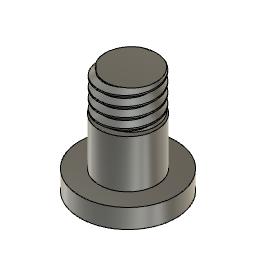
axle wheel right rear (Autodesk Fusion 360 design; units mm, degrees)
Autodesk Fusion 360 part; units mm, degrees
mesh "Mesh1" [no effect] in component "axle wheel right rear"
sketch "axle wheel right rear" plane through (0, 0, 0) normal (0, 0, 1) x (1, 0, 0) in component "axle wheel right rear"
  circle A0 centre (0, 0) radius 5
  circle A1 centre (0, 0) radius 3.0008
  constraint concentric A0 A1
extrude "Extrude1" add sketch "axle wheel right rear" along normal blind 2 contours A0 | A1 makes body 1 in component "axle wheel right rear"
extrude "Extrude2" add sketch "axle wheel right rear" along normal blind 7 contours A1 bodies 1 in component "axle wheel right rear"
extrude "Extrude3" add 1 faces at (0.1785, 0.782, 7) along direction (0, 0, 1) blind 4 separate body on bodies 1 makes body 2 in component "axle wheel right rear"
thread "Thread1" "ISO Metric profile 6.0 M6x1 6g" major diameter 5.884 minor diameter 4.7435 pitch 1 angle 60 modelled right hand crest width 0.1444 on face at (2.997, -0.1496, 9.6667) crest through (2.942, 0, 6.75) on bodies 2 in component "axle wheel right rear"
combine "Combine1" operation add target body 1 tool bodies 2 in component "axle wheel right rear"
component "axle wheel right rear" placed x (1, 0, 0) y (0, 1, 0) z (0, 0, 1) at (0, 0, 0)
named bodies: "axle wheel right rear"
